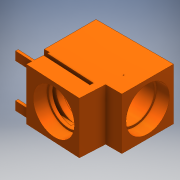
# Autodesk Inventor part: Trappe Lancement 2
Saved by Autodesk Inventor 2016 SP1 (Build 200210100, 210)
## iProperties
Created: 2017-05-09
Part Number: Trappe Lancement 2
Material: Générique
Document SubType Name: Modeling
Designer: dimercur
Density: 1 g/cm^3
Appearance: Lisse - Orange clair
Author: dimercur
Autodesk Inventor part; units mm, degrees
ref_plane "YZ Plane" through (0, 0, 0) normal (1, 0, 0) x (0, 1, 0)
ref_plane "XZ Plane" through (0, 0, 0) normal (0, 1, 0) x (-1, 0, 0)
sketch "Esquisse1" plane through (0, 0, 0) normal (0, 1, 0) x (-1, 0, 0)
  line L0 (45, 30) -> (-45, 30)
  line L1 (-45, 30) -> (-45, -30)
  line L2 (-45, -30) -> (45, -30)
  line L3 (45, -30) -> (45, 30)
  point P0 (0, 0)
  dimension "d0" = 60
  dimension "d1" = 90
  dimension "d2" = 30
  dimension "d3" = 45
  constraints: 8 end point, 2 parallel, 1 horizontal, 1 perpendicular
  measures "d0" distance of L2.end L0.start
  measures "d1" distance of L0.start L0.end
  measures "d2" vertical distance of point (0, 0) L0.start
  measures "d3" horizontal distance of point (0, 0) L0.start
extrude "Extrusion1" add sketch "Esquisse1" along normal blind 60
sketch "Esquisse3" plane through (45, 0, 30) normal (1, 0, 0) x (0, 0, -1)
  circle A0 centre (30, 30) radius 23
  line L0 (0, 0) -> (0, 60) projected
  point P0 (30, 0)
  dimension "d7" = 30
  dimension "d8" = 30
  dimension "d9" = 46
  constraints: 1 centre point
  measures "d7" distance of point (30, 0) A0.centre
  measures "d8" distance from line of L0 A0.centre
  measures "d9" diameter of A0
extrude "Extrusion2" cut sketch "Esquisse3" against normal through all
sketch "Esquisse4" plane through (45, 0, 30) normal (1, 0, 0) x (0, 0, -1)
  circle A0 centre (30, 30) radius 25.25
  circle A1 centre (30, 30) radius 23 projected
  point P0 (30, 0)
  dimension "d12" = 50.5
  constraints: 1 centre point, 1 concentric
  measures "d12" diameter of A0
extrude "Extrusion3" cut sketch "Esquisse4" against normal blind 15
sketch "Esquisse5" plane through (-45, 0, -30) normal (-1, 0, 0) x (0, 0, 1)
  circle A0 centre (30, 30) radius 25.25
  circle A1 centre (30, 30) radius 23 projected
  point P0 (30, 0)
  dimension "d15" = 50.5
  constraints: 1 centre point, 1 concentric
  measures "d15" diameter of A0
extrude "Extrusion4" cut sketch "Esquisse5" against normal blind 15
sketch "Esquisse6" plane through (0, 0, 0) normal (0, -1, 0) x (1, 0, 0)
  circle A0 centre (-5, 0) radius 23
  point P0 (0, 0)
  dimension "d18" = 46
  dimension "d19" = 5
  constraints: 1 centre point
  measures "d18" diameter of A0
  measures "d19" distance of point (0, 0) A0.centre
extrude "Extrusion5" cut sketch "Esquisse6" against normal blind 30
sketch "Esquisse7" plane through (-45, 0, 30) normal (0, 0, 1) x (1, 0, 0)
  circle A0 centre (72, 20) radius 0.5
  line L0 (90, 0) -> (90, 60) projected
  line L1 (0, 60) -> (90, 60) projected
  point P0 (45, 0)
  dimension "d22" = 1
  dimension "d23" = 18
  dimension "d24" = 40
  constraints: 1 centre point
  measures "d22" diameter of A0
  measures "d23" distance from line of L0 A0.centre
  measures "d24" distance from line of L1 A0.centre
extrude "Extrusion6" cut sketch "Esquisse7" against normal through all
sketch "Esquisse8" plane through (-45, 0, -30) normal (-1, 0, 0) x (0, 0, 1)
  line L0 (29.2, 5) -> (30.8, 5)
  line L1 (30.8, 5) -> (30.8, 4.5)
  line L2 (30.8, 4.5) -> (29.2, 4.5)
  line L3 (29.2, 4.5) -> (29.2, 5)
  line L4 (0, 0) -> (60, 0) projected
  point P0 (30, 0)
  dimension "d27" = 0.5
  dimension "d28" = 1.6
  dimension "d29" = 0.8
  dimension "d30" = 4.5
  constraints: 8 end point, 2 parallel, 1 horizontal, 1 perpendicular
  measures "d27" distance of L2.end L0.start
  measures "d28" distance of L1.end L2.end
  measures "d29" horizontal distance of point (30, 0) L2.end
  measures "d30" distance between parallel lines of L4 L2
extrude "Extrusion7" cut sketch "Esquisse8" against normal blind 1
ref_plane "Plan de construction2" through (45, 0, -30) normal (-0.0528447, -0.9986027, 0) x (0, 0, 1)
sketch "Esquisse9" plane through (45, 0, -30) normal (-0.0528447, -0.9986027, 0) x (0, 0, 1)
  line L0 (0, 83.874247) -> (60, 83.874247)
  line L1 (60, 83.874247) -> (60, 18.874247)
  line L2 (60, 18.874247) -> (0, 18.874247)
  line L3 (0, 18.874247) -> (0, 83.874247)
  line L4 (60, 89.874247) -> (60, 93.044928)
  line L5 (0, 89.874247) -> (60, 89.874247)
  point P0 (30, 44.937123)
  dimension "d33" = 60
  dimension "d34" = 0
  dimension "d35" = 65
  dimension "d36" = 6
  constraints: 8 end point, 2 parallel, 1 horizontal, 1 perpendicular
  measures "d33" distance of L0.end L0.start
  measures "d34" distance from line of L4 L0.end
  measures "d35" distance of L2.end L0.start
  measures "d36" distance from line of L5 L0.start
extrude "Extrusion8" add sketch "Esquisse9" along normal blind 30
sketch "Esquisse11" plane through (45, 0, -30) normal (0.0528447, 0.9986027, 0) x (0.9986027, -0.0528447, 0)
  circle A0 centre (-50.069961, -30) radius 23
  ellipse E0 centre (-50.069961, -30) end of major axis (-73.102142, -30) minor radius 23
  point P0 (-44.937123, -30)
  dimension "d39" = 46
  constraints: 1 centre point, 2 other
  measures "d39" diameter of A0
sketch "Esquisse11 outline for Extrusion9" plane through (45, 0, -30) normal (0.0528447, 0.9986027, 0) x (0.9986027, -0.0528447, 0)
  circle A0 centre (-50.069961, -30) radius 23
extrude "Extrusion9" cut sketch "Esquisse11 outline for Extrusion9" against normal blind 30
sketch "Esquisse13" plane through (43.414659, -29.958082, -30) normal (-0.0528447, -0.9986027, 0) x (0.9986027, -0.0528447, 0)
  circle A0 centre (-50.069961, 30) radius 25.25
  circle A1 centre (-50.069961, 30) radius 23
  point P0 (-44.937123, 30)
  dimension "d42" = 50.5
  constraints: 1 centre point, 1 concentric
  measures "d42" diameter of A0
extrude "Extrusion10" cut sketch "Esquisse13" against normal blind 15
sketch "Esquisse15" plane through (-38.991605, 0, -30) normal (-0.9986027, 0.0528447, 0) x (0, 0, 1)
  line L0 (60, 0) -> (60, -25.56149)
  line L1 (60, -6.5) -> (7, -6.5)
  line L2 (7, -6.5) -> (7, -2.5)
  line L3 (7, -2.5) -> (60, -2.5)
  line L4 (60, -2.5) -> (60, -6.5)
  point P0 (30, 2.060499)
  dimension "d45" = 53
  dimension "d46" = 4
  dimension "d47" = 2.5
  constraints: 8 end point, 2 parallel, 1 horizontal, 1 perpendicular, 1 point on line
  measures "d45" distance of L1.start L1.end
  measures "d46" distance between parallel lines of L1 L3
  measures "d47" distance from line of L0.start L3
extrude "Extrusion11" cut sketch "Esquisse15" against normal blind 33.8
sketch "Esquisse16" plane through (-38.991605, 0, -30) normal (-0.9986027, 0.0528447, 0) x (0, 0, 1)
  line L0 (60, -2.5) -> (60, -6.5) projected
  line L1 (7, -2.5) -> (60, -2.5) projected
  line L2 (60, -6.5) -> (30, -6.5)
  line L3 (30, -6.5) -> (30, -2.5)
  line L4 (30, -2.5) -> (60, -2.5)
  line L5 (60, -2.5) -> (60, -6.5)
  point P0 (30, 2.060499)
  dimension "d50" = 30
  constraints: 8 end point, 2 parallel, 1 horizontal, 1 perpendicular, 1 point on line
  measures "d50" distance of L0.end L2.end
extrude "Extrusion12" cut sketch "Esquisse16" against normal blind 56.805
sketch "Esquisse17" plane through (-38.991605, 0, -30) normal (-0.9986027, 0.0528447, 0) x (0, 0, 1)
  line L0 (50.15, -19.5) -> (60, -19.5)
  line L1 (60, -19.5) -> (60, -16.5)
  line L2 (60, -16.5) -> (50.15, -16.5)
  line L3 (50.15, -16.5) -> (50.15, -19.5)
  line L4 (0, -19.5) -> (9.85, -19.5)
  line L5 (9.85, -19.5) -> (9.85, -16.5)
  line L6 (9.85, -16.5) -> (0, -16.5)
  line L7 (0, -16.5) -> (0, -19.5)
  line L8 (60, 3.439711) -> (60, -25.56149)
  line L9 (60, -6.5) -> (7, -6.5)
  line L10 (0, 0) -> (0, -25.56149)
  point P0 (30, 2.060499)
  dimension "d53" = 3
  dimension "d54" = 3
  dimension "d55" = 0
  dimension "d56" = 40.3
  dimension "d57" = 13
  dimension "d58" = 13
  dimension "d60" = 0
  constraints: 16 end point, 4 parallel, 2 horizontal, 2 perpendicular, 1 collinear
  measures "d53" distance between parallel lines of L6 L4
  measures "d54" distance between parallel lines of L2 L0
  measures "d55" distance between parallel lines of L8 L1
  measures "d56" distance between parallel lines of L3 L5
  measures "d57" distance between parallel lines of L4 L9
  measures "d58" distance between parallel lines of L9 L0
  measures "d60" distance between parallel lines of L10 L7
extrude "Extrusion13" add sketch "Esquisse17" along normal blind 20
equation "\"d2\" = 0.5 * d0"
equation "\"d3\" = 0.5 * d1"
equation "\"d29\" = 0.5 * d28"
equation "\"d58\" = d57"
